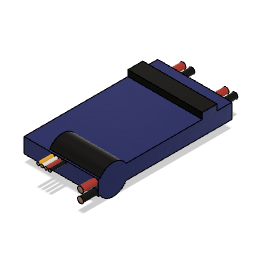
_2s3s ESC.47fdbf37-be1d-40df-9123-f31ac0c2bed0 (Autodesk Fusion 360 design; units mm, degrees)
Autodesk Fusion 360 part; units mm, degrees
note: some values were not read from the file. Set by a fixed rule: which sketch regions a step uses.
sketch "Sketch1" plane through (0, 0, 0) normal (1, 0, 0) x (0, 0, -1)
  line L0 (45, 0) -> (45, 5)
  line L1 (0, 5) -> (0, 0)
  line L2 (35, 5) -> (35, 7)
  line L3 (35, 7) -> (39.9958, 7)
  line L4 (39.9958, 7) -> (39.9958, 5)
  line L5 (35, 5) -> (0, 5)
  line L6 (0, 0) -> (45, 0)
  line L7 (45, 5) -> (39.9958, 5)
  arc A0 (0.6699, 0) -> (9.3301, 0) centre (5, 2.5) ccw
  arc A1 (9.3301, 5) -> (0.6699, 5) centre (5, 2.5) ccw
  dimension "d1" = 45
  constraint horizontal L6
  constraint vertical L0
  constraint horizontal L7
  constraint vertical L1
  constraint coincident L1.end L6.start
  constraint tangent L1 A0
  constraint vertical L2
  constraint horizontal L3
  constraint vertical L4
  constraint collinear L5 L7
  constraint coincident L6 A0.end
  constraint coincident L5 A1.start
  constraint concentric A0 A1
  measures "d1" distance of L1.end L0.start
extrude "Extrude1" add sketch "Sketch1" along normal blind 25 contours L0 L1 L2 L3 L4 L5 L6 L7 makes body 1
cylinder "CylinderPrimitive1" add diameter 2 height 5 placed x (0, 1, 0) y (1, 0, 0) z (0, 0, -1) at (22.5, 2.5, -45) separate body makes body 2
copy_body "CopyPasteBodies1" bodies 2 makes body 3
move_body "Move1" bodies 3 to x (1, 0, 0) y (0, 1, 0) z (0, 0, 1) at (-3, 0, 0)
move_body "Move2" bodies 2 3 to x (1, 0, 0) y (0, 1, 0) z (0, 0, 1) at (-1.5, 0, 0)
copy_body "CopyPasteBodies2" bodies 2 3 makes body 4 makes body 5
move_body "Move3" bodies 4 5 to x (1, 0, 0) y (0, 1, 0) z (0, 0, 1) at (-14.5, 0, 0)
copy_body "CopyPasteBodies3" bodies 2 3 makes body 6 makes body 7
move_body "Move4" bodies 6 7 to x (0, -1, 0) y (1, 0, 0) z (0, 0, 1) at (21.5, 22, 50)
extrude "Extrude2" add sketch "Sketch1" along normal blind 17 from surface at 8 contours L6 A0 | L5 A1 bodies 1
cylinder "CylinderPrimitive2" add diameter 1 height 5 placed x (1, 0, 0) y (0, 1, 0) z (0, 0, 1) at (13.648, 4.4232, 0) separate body makes body 8
copy_body "CopyPasteBodies4" bodies 8 makes body 9
move_body "Move5" bodies 9 to x (1, 0, 0) y (0, 1, 0) z (0, 0, 1) at (-1.3, 0, 0)
copy_body "CopyPasteBodies5" bodies 8 9 makes body 10 makes body 11
move_body "Move6" bodies 10 11 to x (1, 0, 0) y (0, 1, 0) z (0, 0, 1) at (-2.6, 0, 0)
